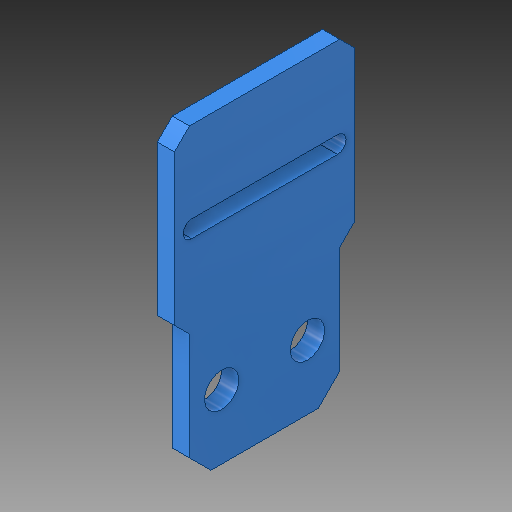
# Autodesk Inventor part: КВ33.044.002 - Держатель катка
Saved by Autodesk Inventor 2019 (Build 230136000, 136)
## iProperties
Created: 2019-07-16
Part Number: КВ33.044.002 - Держатель катка
Material: Пластик АБС
Document SubType Name: Modeling
Designer: user
Density: 1.06 g/cm^3
Appearance: Голубой
Mass: 10.6653 g
Surface Area: 64.099 cm^2
Volume: 10.0616 cm^3
Author: user
Autodesk Inventor part; units mm, degrees
ref_plane "YZ Plane" through (0, 0, 0) normal (1, 0, 0) x (0, 1, 0)
ref_plane "XZ Plane" through (0, 0, 0) normal (0, 1, 0) x (-1, 0, 0)
ref_plane "XY Plane" through (0, 0, 0) normal (0, 0, 1) x (1, 0, 0)
sketch "Эскиз1" plane through (0, 0, 0) normal (1, 0, 0) x (0, 1, 0)
  line L0 (-17.5, 21) -> (-21, 17.5)
  line L1 (-21, 17.5) -> (-21, -17.5)
  line L2 (-21, -17.5) -> (-17.5, -21)
  line L3 (-17.5, -21) -> (17.5, -21)
  line L4 (17.5, -21) -> (21, -17.5)
  line L5 (21, -17.5) -> (21, 17.5)
  line L6 (21, 17.5) -> (17.5, 21)
  line L7 (17.5, 21) -> (-17.5, 21)
  line L8 (-21, 17.5) -> (-51, 17.5)
  line L9 (-51, 17.5) -> (-51, -17.5)
  line L10 (-51, -17.5) -> (-21, -17.5)
  line L11 (-21, -17.5) -> (-21, 17.5)
  line L12 (-51, 0) -> (-36, 0)
  line L13 (-36, 0) -> (-36, 10)
  line L14 (-36, 10) -> (-36, -10)
  circle A0 centre (-36, 10) radius 4
  circle A1 centre (-36, -10) radius 4
  line L15 (0, 17) -> (0, -17) construction
  line L16 (-2, 17) -> (-2, -17)
  line L17 (2, -17) -> (2, 17)
  arc A2 (2, 17) -> (-2, 17) centre (0, 17) ccw
  arc A3 (-2, -17) -> (2, -17) centre (0, -17) ccw
  point P0 (0, 0)
  point P1 (0, 0)
  point P2 (0, 0)
  dimension "d0" = 30
  dimension "d1" = 15
  dimension "d2" = 10
  dimension "d3" = 20
  dimension "d4" = 8
  dimension "d5" = 8
  dimension "d12" = 17
  dimension "d13" = 4
  constraints: 38 end point, 4 centre point, 4 point on circle, 4 tangent, 3 parallel, 2 coincident, 2 horizontal, 2 midpoint, 2 perpendicular, 1 point on line, 1 vertical
  measures "d0" distance of L10.end L9.end
  measures "d1" distance of L12.start L12.end
  measures "d2" distance of L12.end L13.end
  measures "d3" distance of L13.end L14.end
  measures "d4" diameter of A0
  measures "d5" diameter of A1
  measures "d12" distance of point (0, 0) L15.end
  measures "d13" diameter of A3
extrude "Выдавливание1" add sketch "Эскиз1" along normal blind 4
chamfer "Фаска1" distance 5 angle 45 2 edges at (2, -51, 17.5) (2, -51, -17.5)
